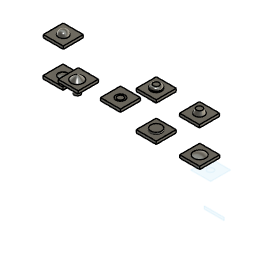
RIVETS_TYPES OF RIVET HEADS (Autodesk Fusion 360 design; units mm, degrees)
Autodesk Fusion 360 part; units mm, degrees
note: some values were not read from the file. Chosen so that the rebuilt part matches the saved one: that a step has no effect; which pieces of a blend or face edit are solid.
sketch "Sketch1" plane through (0, 0, 0) normal (0, 1, 0) x (1, 0, 0)
  line L0 (-150, 0) -> (-150, -25)
  line L1 (-150, -25) -> (-142.5, -25)
  line L2 (-142.5, -25) -> (-142.5, 0)
  line L3 (-142.5, 0) -> (-150, 0)
  line L4 (-150, -25) -> (-138, -25)
  line L5 (-150, -25) -> (-150, -37)
  arc A0 (-150, -37) -> (-138, -25) centre (-150, -25) ccw
  dimension "d2" = 7.5
  dimension "d3" = 12
  dimension "d4" = 12
  constraint perpendicular L0 L1
  constraint perpendicular L1 L2
  constraint perpendicular L2 L3
  constraint perpendicular L0 L4
  constraint perpendicular L4 L5
  measures "d2" distance of L0.end L1.end
  measures "d3" distance of L0.end L4.end
  measures "d4" distance of L0.end L5.end
sketch "Sketch2" plane through (0, 0, 0) normal (0, 1, 0) x (1, 0, 0)
revolve "Revolve1" add sketch "Sketch1" angle 360 about axis through (-150, 0, 0) along (0, 0, 1) makes body 1
sketch "Sketch3" plane through (0, 0, 0) normal (0, 0, 1) x (1, 0, 0)
  line L0 (-225, 25) -> (-175, 25)
  line L1 (-175, 25) -> (-175, -25)
  line L2 (-175, -25) -> (-225, -25)
  line L3 (-225, -25) -> (-225, 25)
  constraint horizontal L0
  constraint vertical L1
  constraint horizontal L2
  constraint vertical L3
extrude "Extrude1" add sketch "Sketch3" along normal blind 20 separate body makes body 2
sketch "Sketch4" plane through (0, 0, 20) normal (0, 0, 1) x (-1, 0, 0)
  line L0 (225, 25) -> (175, 25)
  line L1 (175, 25) -> (175, -25)
  line L2 (175, -25) -> (225, -25)
  line L3 (225, -25) -> (225, 25)
  circle A0 centre (200, 0) radius 7.5
  dimension "d11" = 15
  measures "d11" diameter of A0
extrude "Extrude2" cut sketch "Sketch4" against normal blind 25 contours A0 bodies 2
sketch "Sketch5" plane through (0, 0, 0) normal (0, 1, 0) x (1, 0, 0)
copy_body "CopyPasteBodies1" bodies 2 makes body 3
move_body "Move1" bodies 3 to x (1, 0, 0) y (0, 1, 0) z (0, 0, 1) at (100, 0, 5)
sketch "Sketch6" plane through (0, 0, 0) normal (1, 0, 0) x (0, 1, 0)
sketch "Sketch7" plane through (0, 0, 0) normal (0, 1, 0) x (1, 0, 0)
copy_body "CopyPasteBodies2" bodies 2 makes body 4
move_body "Move2" bodies 4 to x (1, 0, 0) y (0, 1, 0) z (0, 0, 1) at (190.5162, 0, 79.1752)
copy_body "CopyPasteBodies3" bodies 2 makes body 5
move_body "Move3" bodies 5 to x (1, 0, 0) y (0, 1, 0) z (0, 0, 1) at (319.278, 0, 10.6767)
copy_body "CopyPasteBodies4" bodies 2 makes body 6
move_body "Move4" bodies 6 to x (1, 0, 0) y (0, 1, 0) z (0, 0, 1) at (-76.8243, 0, -102.1102)
copy_body "CopyPasteBodies5" bodies 2 makes body 7
move_body "Move5" bodies 7 to x (1, 0, 0) y (0, 1, 0) z (0, 0, 1) at (51.4675, 0, -105.8947)
copy_body "CopyPasteBodies6" bodies 2 makes body 8
move_body "Move6" bodies 8 to x (1, 0, 0) y (0, 1, 0) z (0, 0, 1) at (328.4569, 25, -75.158)
copy_body "CopyPasteBodies7" bodies 2 makes body 9
move_body "Move7" bodies 9 to x (1, 0, 0) y (0, 1, 0) z (0, 0, 1) at (190, 0, -90)
move_body "Move8" bodies 1 to x (1, 0, 0) y (0, 1, 0) z (0, 0, 1) at (-50, 0, -5)
sketch "Sketch8" plane through (0, 0, 0) normal (0, 1, 0) x (1, 0, 0)
move_body "Move9" bodies 2 to x (1, 0, 0) y (0, 1, 0) z (0, 0, 1) at (50, 25, 90)
move_body "Move10" bodies 2 to x (1, 0, 0) y (0, 1, 0) z (0, 0, 1) at (-50, -25, -90)
sketch "Sketch9" plane through (0, 0, 0) normal (0, 1, 0) x (1, 0, 0)
move_face "OffsetFaces1" offset -13 1 faces at (-200.1868, -19.1597, 0) on bodies 2
move_face "OffsetFaces2" offset -13 7 faces at (-277.0111, -19.1597, -102.1102) (-10.1868, -19.1597, -90) (128.2701, 5.8403, -75.158) (119.0912, -19.1597, 10.6767) (-148.7193, -19.1597, -105.8947) (-9.6706, -19.1597, 79.1752) (-100.1868, -19.1597, 5) on bodies 3 4 5 6 7 8 9
sketch "Sketch10" plane through (0, 0, 0) normal (0, 1, 0) x (1, 0, 0)
  line L0 (-25, -25) -> (-25, 0)
  line L1 (-25, 0) -> (-17.5, 0)
  line L2 (-17.5, 0) -> (-17.5, -25)
  line L3 (-17.5, -25) -> (-25, -25)
  line L4 (-25, -25) -> (-21.25, -25)
  dimension "d25" = 7.5
  dimension "d26" = 3.75
  constraint vertical L0
  constraint perpendicular L0 L1
  constraint perpendicular L1 L2
  constraint perpendicular L0 L3
  constraint midpoint L3 L4.end
  measures "d25" distance of L0.end L1.end
  measures "d26" distance of L0.start L4.end
revolve "Revolve2" add sketch "Sketch10" angle 360 about axis through (-25, 0, 25) along (0, 0, -1) separate body makes body 10
pattern_linear "R-Pattern1" count 3 spacing 45 along (1, 0, 0) of bodies 10 makes body 11 at (27.4907, 0.3738, 8.3333) makes body 12 at (72.4907, 0.3738, 8.3333)
form "Form1" [no effect]
pattern_linear "R-Pattern2" count 4 spacing 33.3333 along (1, 0, 0) of bodies 12 makes body 13 at (105.824, 0.3738, 8.3333) makes body 14 at (139.1573, 0.3738, 8.3333) makes body 15 at (172.4907, 0.3738, 8.3333)
move_body "Move11" bodies 10 to x (1, 0, 0) y (0, 1, 0) z (0, 0, 1) at (-75, 0, 0)
sketch "Sketch11" plane through (0, 0, 25) normal (0, 0, 1) x (-1, 0, 0)
  circle A0 centre (100, 0) radius 7.5
  circle A1 centre (100, 0) radius 15
  dimension "d36" = 30
  constraint concentric A0 A1
  measures "d36" diameter of A1
extrude "Extrude3" add sketch "Sketch11" along normal blind 3.75 contours A0 | A1 bodies 3 10
sketch "Sketch12" plane through (0, 0, 0) normal (0, 1, 0) x (1, 0, 0)
  line L0 (-35, -1) -> (-20, -1)
  line L1 (-35, -1) -> (-35, -4.75)
  arc A0 (-35, -4.75) -> (-20, -1) centre (-35, 27.125) ccw
  dimension "d41" = 3.75
  constraint horizontal L0
  constraint perpendicular L0 L1
  measures "d41" distance of L0.start L1.end
revolve "Revolve3" add sketch "Sketch12" angle 360 about axis through (-35, 0, 1) along (0, 0, 1) separate body makes body 16
move_body "Move12" bodies 16 to x (1, 0, 0) y (0, 1, 0) z (0, 0, 1) at (55, 0, 24)
sketch "Sketch13" plane through (0, 0, 0) normal (0, 1, 0) x (1, 0, 0)
  line L0 (-50.9097, 33.3834) -> (-50.9097, 22.8834)
  line L1 (-50.9097, 22.8834) -> (-43.4097, 22.8834)
  line L2 (-50.9097, 33.3834) -> (-38.9097, 33.3834)
  line L3 (-43.4097, 22.8834) -> (-38.9097, 33.3834)
  dimension "d43" = 10.5
  dimension "d44" = 7.5
  dimension "d45" = 12
  constraint vertical L0
  constraint perpendicular L0 L1
  constraint perpendicular L0 L2
  measures "d43" distance of L0.start L0.end
  measures "d44" distance of L0.end L1.end
  measures "d45" distance of L0.start L2.end
revolve "Revolve4" add sketch "Sketch13" angle 360 about axis through (-50.9097, 0, -33.3834) along (0, 0, 1) separate body makes body 17
move_body "Move13" bodies 17 to x (1, 0, 0) y (0, 1, 0) z (0, 0, 1) at (115.9097, 0, 58.3834)
sketch "Sketch14" plane through (0, 0, 0) normal (0, 1, 0) x (1, 0, 0)
  line L0 (100, -100) -> (113.2, -100)
  line L1 (100, -100) -> (100, -109)
  line L2 (100, -109) -> (113.2, -109)
  line L3 (113.2, -109) -> (113.2, -100)
  dimension "d47" = 13.2
  dimension "d48" = 9
  constraint horizontal L0
  constraint perpendicular L0 L1
  constraint perpendicular L1 L2
  constraint perpendicular L2 L3
  measures "d47" distance of L0.start L0.end
  measures "d48" distance of L0.start L1.end
revolve "Revolve5" add sketch "Sketch14" angle 360 about axis through (100, 0, 100) along (0, 0, 1) separate body makes body 18
fillet "Fillet1" radius 6 1 edges at (87.6933, -4.7733, 109) on bodies 18
move_body "Move14" bodies 18 to x (1, 0, 0) y (0, 1, 0) z (0, 0, 1) at (65, 0, -75)
move_body "Move15" bodies 16 11 to x (1, 0, 0) y (0, 1, 0) z (0, 0, 1) at (-30, 0, -95)
move_body "Move16" bodies 17 12 to x (1, 0, 0) y (0, 1, 0) z (0, 0, 1) at (-213.5325, 0, -110.8947)
move_body "Move17" bodies 18 15 to x (1, 0, 0) y (0, 1, 0) z (0, 0, 1) at (-441.8243, 0, -107.1102)
delete_face "DeleteFace1" 1 faces at (-114.9255, 1.4935, 27.5) on bodies 3
sketch "Sketch15" plane through (0, -25, 0) normal (0, -1, 0) x (1, 0, 0)
  line L0 (-125, 18) -> (-75, 18)
  line L1 (-75, 18) -> (-75, 25)
  line L2 (-75, 25) -> (-125, 25)
  line L3 (-125, 25) -> (-125, 18)
  line L4 (-35, 15) -> (-35, 16.875)
  line L5 (-35, 15) -> (-35, 13.125)
  line L6 (-35, 16.875) -> (-21.4455, 16.875)
  line L7 (-21.4455, 13.125) -> (-35, 13.125)
  arc A0 (-21.4455, 13.125) -> (-21.4455, 16.875) centre (-21.9388, 15) ccw
  dimension "d53" = 1.875
  dimension "d54" = 1.875
  constraint perpendicular L4 L6
  constraint perpendicular L5 L7
  measures "d53" distance of L4.start L4.end
  measures "d54" distance of L4.start L5.end
revolve "Revolve6" add sketch "Sketch15" angle 360 about axis through (-35, -25, 15) along (0, 0, -1) separate body contours L4 L5 L6 L7 A0 makes body 19
move_body "Move18" bodies 19 to x (1, 0, 0) y (0, 1, 0) z (0, 0, 1) at (-65, 25, 11.875)
sketch "Sketch16" plane through (0, 0, 0) normal (1, 0, 0) x (0, 1, 0)
sketch "Sketch17" plane through (0, -25, 0) normal (0, -1, 0) x (1, 0, 0)
  line L0 (-125, 18) -> (-75, 18)
  line L1 (-75, 18) -> (-75, 25)
  line L2 (-75, 25) -> (-125, 25)
  line L3 (-125, 25) -> (-125, 18)
  line L4 (17.771, 24.6922) -> (17.771, 0)
  line L5 (17.771, 0) -> (25.271, 0)
  line L6 (25.271, 0) -> (25.271, 24.6922)
  line L7 (25.271, 24.6922) -> (17.771, 24.6922)
  line L8 (17.771, 24.6922) -> (17.771, 28.4422)
  line L9 (17.771, 28.4422) -> (29.021, 28.4422)
  line L10 (29.021, 28.4422) -> (25.271, 24.6922)
  dimension "d56" = 7.5
  dimension "d57" = 3.75
  dimension "d58" = 11.25
  constraint vertical L4
  constraint perpendicular L4 L5
  constraint perpendicular L5 L6
  constraint perpendicular L4 L7
  constraint perpendicular L7 L8
  constraint perpendicular L8 L9
  measures "d56" distance of L4.end L5.end
  measures "d57" distance of L4.start L8.end
  measures "d58" distance of L8.end L9.end
revolve "Revolve7" add sketch "Sketch17" angle 360 about axis through (17.771, -25, 24.6922) along (0, 0, -1) separate body contours L4 L5 L6 L7 | L7 L8 L9 L10 makes body 20
sketch "Sketch18" plane through (0, 0, 0) normal (0, 1, 0) x (1, 0, 0)
sketch "Sketch19" plane through (0, 0, 0) normal (0, 1, 0) x (1, 0, 0)
sketch "Sketch20" plane through (0, 0, 0) normal (0, 1, 0) x (1, 0, 0)
sketch "Sketch21" plane through (0, -25, 0) normal (0, -1, 0) x (1, 0, 0)
sketch "Sketch22" plane through (0, 0, 0) normal (0, -1, 0) x (1, 0, 0)
  line L0 (103.4569, -62.158) -> (153.4569, -62.158)
  line L1 (153.4569, -62.158) -> (153.4569, -55.158)
  line L2 (153.4569, -55.158) -> (103.4569, -55.158)
  line L3 (103.4569, -55.158) -> (103.4569, -62.158)
ref_plane "WorkPlane1" through (128.4569, 25, -58.658) normal (0, 1, 0) x (-1, 0, 0)
sketch "Sketch23" plane through (0, 25, 0) normal (0, 1, 0) x (1, 0, 0)
  line L0 (103.4569, 62.158) -> (103.4569, 55.158)
  line L1 (153.4569, 62.158) -> (153.4569, 55.158)
  line L2 (103.4569, 62.158) -> (153.4569, 62.158)
  line L3 (103.4569, 55.158) -> (153.4569, 55.158)
  line L4 (103.4569, 55.158) -> (128.4569, 55.158)
  line L5 (128.4569, 55.158) -> (128.4569, 70)
  line L6 (128.4569, 70) -> (135.9569, 70)
  line L7 (128.4569, 55.158) -> (139.7069, 55.158)
  line L8 (128.4569, 55.158) -> (128.4569, 58.908)
  line L9 (128.4569, 58.908) -> (135.9569, 58.908)
  line L10 (135.9569, 58.908) -> (139.7069, 55.158)
  line L11 (135.9569, 58.908) -> (135.9569, 70)
  dimension "d70" = 7.5
  dimension "d71" = 11.25
  dimension "d72" = 3.75
  constraint coincident L0.end L3.start
  constraint midpoint L3 L4.end
  constraint perpendicular L3 L5
  constraint perpendicular L5 L6
  constraint perpendicular L5 L7
  constraint perpendicular L7 L8
  constraint perpendicular L5 L9
  constraint perpendicular L6 L11
  measures "d70" distance of L5.end L6.end
  measures "d71" distance of L4.end L7.end
  measures "d72" distance of L4.end L8.end
revolve "Revolve8" add sketch "Sketch23" angle 360 about axis through (128.4569, 25, -55.158) along (0, 0, -1) separate body contours L2 L5 L6 L11 | L2 L5 L9 L11 | L3 L5 L7 L8 L9 L10 makes body 21
sketch "Sketch24" plane through (0, 0, 0) normal (0, 1, 0) x (1, 0, 0)
sketch "Sketch25" plane through (0, 0, 28.4422) normal (0, 0, 1) x (-1, 0, 0)
  circle A0 centre (-17.771, 25) radius 11.25
  circle A1 centre (-17.771, 25) radius 11.25
  constraint concentric A0 A1
extrude "Extrude4" cut sketch "Sketch25" against normal blind 40 bodies 20
sketch "Sketch26" plane through (0, 0, 99.1752) normal (0, 0, 1) x (-1, 0, 0)
sketch "Sketch27" plane through (0, 0, 99.1752) normal (0, 0, 1) x (-1, 0, 0)
sketch "Sketch28" plane through (15.5162, 0, 0) normal (1, 0, 0) x (0, 1, 0)
sketch "Sketch29" plane through (0, 0, 99.1752) normal (0, 0, 1) x (-1, 0, 0)
  circle A0 centre (9.4838, 0) radius 7.5
  line L0 (34.4838, 25) -> (-15.5162, 25)
  line L1 (-15.5162, 25) -> (-15.5162, -25)
  line L2 (-15.5162, -25) -> (34.4838, -25)
  line L3 (34.4838, -25) -> (34.4838, 25)
  line L4 (-15.5162, 25) -> (37, 25)
  line L5 (37, 25) -> (37, -27)
  line L6 (37, -27) -> (-15.5162, -27)
  line L7 (-15.5162, -27) -> (-15.5162, 25)
  constraint horizontal L4
  constraint vertical L5
  constraint horizontal L6
  constraint vertical L7
  constraint coincident L0.end L1.start
extrude "Extrude5" cut sketch "Sketch29" against normal blind 17 bodies 4
sketch "Sketch30" plane through (0, 0, 0) normal (0, 1, 0) x (1, 0, 0)
sketch "Sketch31" plane through (0, 0, 0) normal (0, 1, 0) x (1, 0, 0)
move_body "Move19" bodies 13 to x (1, 0, 0) y (0, 1, 0) z (0, 0, 1) at (-136.3143, 0, 91.4819)
move_body "Move20" bodies 14 to x (1, 0, 0) y (0, 1, 0) z (0, 0, 1) at (-101.6667, 0, 87.5)
ref_plane "WorkPlane2" through (119.278, 0, 27.1767) normal (1, 0, 0) x (0, 1, 0)
sketch "Sketch32" plane through (119.278, 0, 0) normal (1, 0, 0) x (0, 1, 0)
sketch "Sketch33" plane through (0, 0, 30.6767) normal (0, 0, 1) x (-1, 0, 0)
  circle A0 centre (-119.278, 0) radius 7.5
  line L0 (-94.278, 25) -> (-144.278, 25)
  line L1 (-144.278, 25) -> (-144.278, -25)
  line L2 (-144.278, -25) -> (-94.278, -25)
  line L3 (-94.278, -25) -> (-94.278, 25)
ref_plane "WorkPlane3" through (119.278, 0, 27.1767) normal (0, 1, 0) x (-1, 0, 0)
sketch "Sketch34" plane through (0, 0, 0) normal (0, 1, 0) x (1, 0, 0)
sketch "Sketch35" plane through (0, 0, 0) normal (0, 1, 0) x (1, 0, 0)
  line L0 (94.278, -23.6767) -> (94.278, -30.6767)
  line L1 (144.278, -23.6767) -> (144.278, -30.6767)
  line L2 (94.278, -23.6767) -> (144.278, -23.6767)
  line L3 (94.278, -30.6767) -> (144.278, -30.6767)
  line L4 (119.278, -30.6767) -> (119.278, -7)
  line L5 (119.278, -7) -> (126.778, -7)
  line L6 (119.278, -30.6767) -> (119.278, -26.9267)
  line L7 (119.278, -26.9267) -> (126.778, -26.9267)
  line L8 (126.778, -26.9267) -> (126.778, -7)
  line L9 (126.778, -26.9267) -> (119.278, -26.9267)
  line L10 (119.278, -30.6767) -> (130.528, -30.6767)
  line L11 (130.528, -30.6767) -> (126.778, -26.9267)
  line L12 (119.278, -30.6767) -> (119.278, -33.6767)
  arc A0 (119.278, -33.6767) -> (130.528, -30.6767) centre (119.278, -11.0829) ccw
  dimension "d79" = 7.5
  dimension "d80" = 3.75
  dimension "d81" = 11.25
  dimension "d83" = 3
  constraint midpoint L3 L4.start
  constraint perpendicular L2 L4
  constraint perpendicular L4 L5
  constraint perpendicular L6 L7
  constraint perpendicular L5 L8
  constraint perpendicular L4 L10
  constraint symmetric L4.start L6 L10.start
  constraint perpendicular L3 L12
  measures "d79" distance of L4.end L5.end
  measures "d80" distance of L4.start L6.end
  measures "d81" distance of L4.start L10.end
  measures "d83" distance of L4.start L12.end
revolve "Revolve9" add sketch "Sketch35" angle 360 about axis through (119.278, 0, 30.6767) along (0, 0, -1) separate body contours L2 L4 L5 L8 | L2 L4 L7 L8 L9 | L3 L4 L6 L7 L9 L10 L11 | L3 L10 L12 A0 makes body 22
sketch "Sketch36" plane through (0, 0, 112.5) normal (0, 0, 1) x (-1, 0, 0)
  circle A0 centre (-30, 0) radius 7.5
  circle A1 centre (-30, 0) radius 7.5
  constraint concentric A0 A1
extrude "Extrude6" cut sketch "Sketch36" against normal blind 20 bodies 14
extrude "Extrude7" cut 1 faces at (29.9022, 1.2462, 92.5) along direction (0, 0, -1) blind 10 on bodies 14 bodies 14
sketch "Sketch37" plane through (0, 0, 116.4819) normal (0, 0, 1) x (-1, 0, 0)
  circle A0 centre (37.981, 0) radius 7.5
  circle A1 centre (37.981, 0) radius 7.5
  constraint concentric A0 A1
extrude "Extrude8" cut sketch "Sketch37" against normal blind 29 bodies 13
sketch "Sketch38" plane through (0, 0, 0) normal (0, 1, 0) x (1, 0, 0)
  line L0 (-50, -150) -> (-50, -120)
  line L1 (-50, -120) -> (-57.5, -120)
  line L2 (-57.5, -120) -> (-50, -120)
  line L3 (-50, -150) -> (-57.5, -150)
  line L4 (-57.5, -150) -> (-57.5, -120)
  line L5 (-50, -150) -> (-65, -150)
  line L6 (-50, -150) -> (-50, -160.5)
  spline S0 degree 2 poles (-50, -160.5) (-53.75, -160.5) (-65, -150) knots 0 0 0 1.851221 1.851221 1.851221 weights 1 1.414214 1
  dimension "d91" = 7.5
  dimension "d92" = 15
  dimension "d93" = 10.5
  constraint vertical L0
  constraint perpendicular L0 L1
  constraint perpendicular L0 L3
  constraint perpendicular L1 L4
  constraint perpendicular L0 L5
  constraint perpendicular L5 L6
  measures "d91" distance of L0.end L1.end
  measures "d92" distance of L0.start L5.end
  measures "d93" distance of L0.start L6.end
revolve "Revolve10" add sketch "Sketch38" angle 360 about axis through (-50, 0, 150) along (0, 0, -1) bodies 4 13 14 20
sketch "Sketch39" plane through (0, 0, 30.6767) normal (0, 0, 1) x (-1, 0, 0)
  line L0 (-140.5918, 103.1656) -> (-90.4829, 103.1656)
  line L1 (-90.4829, 103.1656) -> (-90.4829, 52.5236)
  line L2 (-90.4829, 52.5236) -> (-140.5918, 52.5236)
  line L3 (-140.5918, 52.5236) -> (-140.5918, 103.1656)
  constraint horizontal L0
  constraint vertical L1
  constraint horizontal L2
  constraint vertical L3
extrude "Extrude9" add sketch "Sketch39" along normal blind 7 separate body makes body 23
sketch "Sketch40" plane through (0, 0, 37.6767) normal (0, 0, 1) x (-1, 0, 0)
  line L0 (-140.5918, 52.5236) -> (-90.4829, 52.5236)
  line L1 (-90.4829, 52.5236) -> (-90.4829, 103.1656)
  line L2 (-90.4829, 103.1656) -> (-140.5918, 103.1656)
  line L3 (-140.5918, 103.1656) -> (-140.5918, 52.5236)
  circle A0 centre (-115, 80) radius 15
  dimension "d99" = 30
  measures "d99" diameter of A0
extrude "Extrude10" cut sketch "Sketch40" against normal blind 7 contours A0 bodies 23
move_body "Move21" bodies 4 to x (1, 0, 0) y (0, 1, 0) z (0, 0, 1) at (165, -80, -112.3233)
sketch "Sketch41" plane through (0, 0, 0) normal (0, 1, 0) x (1, 0, 0)
move_body "Move22" bodies 1 2 to x (1, 0, 0) y (0, 1, 0) z (0, 0, 1) at (0, 0, 120)
move_body "Move23" bodies 23 4 to x (1, 0, 0) y (0, 1, 0) z (0, 0, 1) at (-240, 0, 102)
move_body "Move24" bodies 15 18 6 to x (1, 0, 0) y (0, 1, 0) z (0, 0, 1) at (230, 0, 222)
move_body "Move25" bodies 17 7 12 to x (1, 0, 0) y (0, 1, 0) z (0, 0, 1) at (180, 0, 226)
move_body "Move26" bodies 22 5 to x (1, 0, 0) y (0, 1, 0) z (0, 0, 1) at (-320, 0, 20)
move_body "Move27" bodies 8 21 to x (1, 0, 0) y (0, 1, 0) z (0, 0, 1) at (-250, 0, 105)
move_body "Move28" bodies 3 19 to x (1, 0, 0) y (0, 1, 0) z (0, 0, 1) at (53, 0, 25)
move_body "Move29" bodies 11 16 9 to x (1, 0, 0) y (0, 1, 0) z (0, 0, 1) at (42, 0, 120)
sketch "Sketch42" plane through (0, 0, 35) normal (0, 0, -1) x (1, 0, 0)
  circle A0 centre (-121.5431, -25) radius 7.5
  circle A1 centre (-121.5431, -25) radius 7.5
  constraint concentric A0 A1
extrude "Extrude11" add sketch "Sketch42" along normal blind 10 bodies 21
move_body "Move30" bodies 1 2 22 5 to x (1, 0, 0) y (0, 1, 0) z (0, 0, 1) at (-50, 0, 0)
move_body "Move31" bodies 23 4 8 21 to x (1, 0, 0) y (0, 1, 0) z (0, 0, 1) at (-30, 0, 0)
move_body "Move32" bodies 7 12 17 9 16 11 to x (1, 0, 0) y (0, 1, 0) z (0, 0, 1) at (60, 0, 0)
move_body "Move33" bodies 18 6 15 3 19 to x (1, 0, 0) y (0, 1, 0) z (0, 0, 1) at (30, 0, 0)
move_body "Move34" bodies 4 23 8 21 to x (1, 0, 0) y (0, 1, 0) z (0, 0, 1) at (20, 0, 0)
